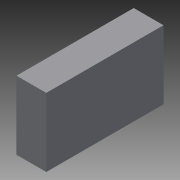
# Autodesk Inventor part: CNC-X-axis- drawer block
Saved by Autodesk Inventor 2015 (Build 190159000, 159)
## iProperties
Created: 2015-03-21
Part Number: CNC-X-axis- drawer block
Material: Generic
Document SubType Name: Modeling
Designer: Bangladesh
Density: 1 g/cm^3
Appearance: Default
Author: Bangladesh
Autodesk Inventor part; units mm, degrees
ref_plane "YZ Plane" through (0, 0, 0) normal (1, 0, 0) x (0, 1, 0)
ref_plane "XZ Plane" through (0, 0, 0) normal (0, 1, 0) x (-1, 0, 0)
ref_plane "XY Plane" through (0, 0, 0) normal (0, 0, 1) x (1, 0, 0)
sketch "Sketch2" plane through (0, 0, 0) normal (0, 0, 1) x (1, 0, 0)
  line L0 (-12.7, 29.21) -> (12.7, 29.21)
  line L1 (12.7, 29.21) -> (12.7, -29.21)
  line L2 (12.7, -29.21) -> (-12.7, -29.21)
  line L3 (-12.7, -29.21) -> (-12.7, 29.21)
  line L4 (-12.7, 29.21) -> (12.7, -29.21) construction
  line L5 (12.7, 29.21) -> (-12.7, -29.21) construction
  point P0 (0, 0)
  dimension "d0" = 25.4
  dimension "d1" = 58.42
  constraints: 12 end point, 2 midpoint, 2 parallel, 1 horizontal, 1 perpendicular
  measures "d0" distance of L1.end L2.end
  measures "d1" distance of L0.end L1.end
extrude "Extrusion1" add sketch "Sketch2" along normal mid plane 100
body "Solid1"
